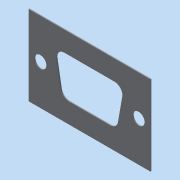
# Autodesk Inventor part: gasketdsub9
Saved by Autodesk Inventor 2016 (Build 200138000, 138)
## iProperties
Created: 2016-10-07
Part Number: gasketdsub9
Material: Generic
Document SubType Name: Modeling
Designer: Zara
Density: 1 g/cm^3
Appearance: Default
Author: Zara
Autodesk Inventor part; units mm, degrees
ref_plane "YZ Plane" through (0, 0, 0) normal (1, 0, 0) x (0, 1, 0)
ref_plane "XZ Plane" through (0, 0, 0) normal (0, 1, 0) x (-1, 0, 0)
ref_plane "XY Plane" through (0, 0, 0) normal (0, 0, 1) x (1, 0, 0)
sketch "Sketch1" plane through (0, 0, 0) normal (0, 0, 1) x (1, 0, 0)
  line L0 (-15.494, -10.16) -> (15.494, -10.16)
  line L1 (15.494, -10.16) -> (15.494, 10.16)
  line L2 (15.494, 10.16) -> (-15.494, 10.16)
  line L3 (-15.494, 10.16) -> (-15.494, -10.16)
  line L4 (-15.494, -10.16) -> (15.494, 10.16) construction
  line L5 (15.494, -10.16) -> (-15.494, 10.16) construction
  line L6 (-6.3834, 5.08) -> (6.3475, 5.08)
  arc A0 (8.3795, 3.048) -> (6.3475, 5.08) centre (6.3475, 3.048) ccw
  line L7 (8.3795, 3.048) -> (7.2424, -3.4009)
  arc A1 (5.2412, -5.08) -> (7.2424, -3.4009) centre (5.2412, -3.048) ccw
  line L8 (5.2412, -5.08) -> (-5.3085, -5.08)
  line L9 (8.3795, 3.048) -> (8.3795, -2.029) construction
  arc A2 (-7.3097, -3.4009) -> (-5.3085, -5.08) centre (-5.3085, -3.048) ccw
  line L10 (-7.3097, -3.4009) -> (-8.3845, 2.6951)
  arc A3 (-6.3834, 5.08) -> (-8.3845, 2.6951) centre (-6.3834, 3.048) ccw
  line L11 (-8.3845, 2.6951) -> (-8.3845, -5.4012) construction
  circle A4 centre (12.4968, 0) radius 1.524
  circle A5 centre (-12.4968, 0) radius 1.524
  point P0 (0, 0)
  dimension "d0" = 30.988
  dimension "d1" = 20.32
  dimension "d2" = 10
  dimension "d4" = 10.16
  dimension "d5" = 10
  dimension "d6" = 7.1095
  dimension "d7" = 5.08
  dimension "d8" = 2.032
  dimension "d9" = 2.032
  dimension "d10" = 2.032
  dimension "d11" = 2.032
  dimension "d12" = 16.764
  dimension "d13" = 24.9936
  dimension "d14" = 3.048
  dimension "d15" = 3.048
  dimension "d16" = 2.9972
  dimension "d17" = 10.16
  dimension "d18" = 10.16
  constraints: 24 end point, 8 point on circle, 8 tangent, 6 centre point, 3 horizontal, 2 midpoint, 2 parallel, 2 vertical, 1 perpendicular
  measures "d0" distance of L1.end L2.end
  measures "d1" distance of L0.end L1.end
  measures "d2" angle of L7 L9
  measures "d4" distance between parallel lines of L6 L8
  measures "d5" angle of L10 L11
  measures "d6" distance from line of L3 L10.end
  measures "d7" distance between parallel lines of L2 L6
  measures "d8" radius of A0
  measures "d9" radius of A3
  measures "d10" radius of A1
  measures "d11" radius of A2
  measures "d12" distance between parallel lines of L11 L9
  measures "d13" distance of A4.centre A5.centre
  measures "d14" diameter of A5
  measures "d15" diameter of A4
  measures "d16" distance from line of L3 A5.centre
  measures "d17" distance from line of L2 A5.centre
  measures "d18" distance from line of L2 A4.centre
extrude "Extrusion1" add sketch "Sketch1" along normal blind 0.254
body "Solid1"
